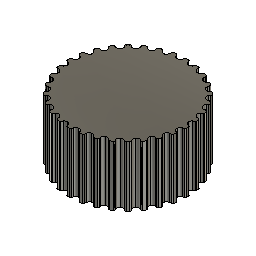
gear_32z (Autodesk Fusion 360 design; units mm, degrees)
Autodesk Fusion 360 part; units mm, degrees
sketch "Sketch1" plane through (0, 0, 0) normal (0, 0, 1) x (1, 0, 0) in component "gt2 pulley"
  circle A0 centre (0, 0) radius 10.1859 construction
  circle A1 centre (0, 0) radius 9.1819 construction
  line L0 (0, 0) -> (0, 10.1859) construction
  line L1 (0, 0) -> (0.9984, 10.1369) construction
  line L2 (0, 0) -> (1.4098, 10.0879) construction
  circle A2 centre (0, 0) radius 9.9319 construction
  arc A3 (0.3759, 9.7867) -> (0.4302, 9.5076) centre (1.3746, 9.8363) ccw
  circle A4 centre (0, 0) radius 9.7819 construction
  arc A5 (0.2295, 9.9293) -> (0, 9.9319) centre (0, 0) ccw
  arc A6 (0.3759, 9.7867) -> (0.2295, 9.9293) centre (0.2261, 9.7793) ccw
  arc A7 (0.4302, 9.5076) -> (0.9, 9.1377) centre (0.9544, 9.69) ccw
  arc A8 (0, 9.9319) -> (-0.2295, 9.9293) centre (0, 0) ccw
  arc A9 (-0.2295, 9.9293) -> (-0.3759, 9.7867) centre (-0.2261, 9.7793) ccw
  arc A10 (-0.4302, 9.5076) -> (-0.3759, 9.7867) centre (-1.3746, 9.8363) ccw
  arc A11 (-0.9002, 9.1377) -> (-0.4302, 9.5076) centre (-0.9544, 9.69) ccw
  arc A12 (0.9, 9.1377) -> (-0.9, 9.1377) centre (0, 0) ccw
  point P0 (1.3746, 9.8363)
  point P1 (0, 9.9319)
  dimension "d18" = 20.3718
  dimension "d19" = 5.625
  dimension "d22" = 1.004
  dimension "d24" = 0.75
  dimension "d26" = 1
  dimension "d27" = 0.15
  dimension "d28" = 0.15
  dimension "d47" = 0.555
  dimension "d52" = 3.812
  constraint coincident A0.centre A1.centre
  constraint coincident A0 L0.end
  constraint vertical L0
  constraint coincident A0 L1.end
  constraint coincident A0 L2.end
  constraint concentric A1 A2
  constraint coincident A1 A7.end
  constraint coincident L1 A7.end
  constraint coincident A2 P0
  constraint coincident L2 P0
  constraint coincident P0 A3.centre
  constraint coincident A2 P1
  constraint coincident L0 P1
  constraint concentric A2 A4
  constraint coincident P1 A5.end
  constraint coincident A4 A6.centre
  constraint coincident A3.start A6.start
  constraint tangent A3 A6
  constraint tangent A3 A7
  constraint symmetric L0 A7.end A12.end
  constraint symmetric L0 A3.start A9.end
  constraint symmetric L0 A3.end A10.start
  constraint symmetric L0 A3 A10
  constraint symmetric L0 A5.start A8.end
  constraint symmetric L0 P1 A5.end
  constraint symmetric L0 A5 A8
  constraint symmetric L0 A6 A9
  constraint symmetric L0 A7 A11
  constraint coincident A1 A11.start
  constraint tangent A1 A7
  constraint coincident L1 A7.centre
  measures "d18" diameter of A0
  measures "d19" angle of L0 L1
  measures "d22" distance of A0 A1
  measures "d24" distance of A1 A2
  measures "d26" radius of A3
  measures "d27" distance of A2 A4
  measures "d28" radius of A6
  measures "d47" radius of A7
extrude "Extrude1" add sketch "Sketch1" along normal blind 10 makes body 1
pattern_circular "C-Pattern1" count 32 over 360 about axis through (0, 0, 1.75) along (0, 0, 1) of bodies 1 makes body 2 at (-1.0991, 9.1159, 6.6667) makes body 3 at (-2.8564, 8.7263, 6.6667) makes body 4 at (-4.504, 8.0014, 6.6667) makes body 5 at (-5.9784, 6.9689, 6.6667) makes body 6 at (-7.5784, 5.1841, 6.6667) makes body 7 at (-8.4442, 3.606, 6.6667) makes body 8 at (-8.9854, 1.8893, 6.6667) makes body 9 at (-9.1551, -0.7007, 6.6667) makes body 10 at (-9.0245, -1.6931, 6.6667) makes body 11 at (-8.7263, -2.8564, 6.6667) makes body 12 at (-7.223, -5.6689, 6.6667) makes body 13 at (-6.9689, -5.9784, 6.6667) makes body 14 at (-4.5038, -8.0015, 6.6667) makes body 15 at (-3.606, -8.4442, 6.6667) makes body 16 at (-1.8893, -8.9854, 6.6667) makes body 17 at (0.7007, -9.1551, 6.6667) makes body 18 at (1.6931, -9.0245, 6.6667) makes body 19 at (2.8564, -8.7263, 6.6667) makes body 20 at (5.1843, -7.5783, 6.6667) makes body 21 at (6.9691, -5.9782, 6.6667) makes body 22 at (7.5784, -5.1841, 6.6667) makes body 23 at (8.1902, -4.1506, 6.6667) makes body 24 at (8.9854, -1.8893, 6.6667) makes body 25 at (9.1551, 0.7007, 6.6667) makes body 26 at (9.1159, 1.0991, 6.6667) makes body 27 at (8.7263, 2.8564, 6.6667) makes body 28 at (7.223, 5.6689, 6.6667) makes body 29 at (6.9689, 5.9784, 6.6667) makes body 30 at (5.1841, 7.5784, 6.6667) makes body 31 at (3.606, 8.4442, 6.6667) makes body 32 at (1.8893, 8.9854, 6.6667)
sketch "Sketch2" plane through (0, 0, 10) normal (0, 0, 1) x (-1, 0, 0)
  arc A0 (-9.672, -1.5406) -> (-9.7832, -1.712) centre (-9.6355, -1.6861) ccw
  arc A1 (-9.7832, -1.712) -> (-9.6937, -2.1622) centre (0, 0) ccw
  arc A2 (-9.6937, -2.1622) -> (-9.5254, -2.278) centre (-9.5473, -2.1296) ccw
  arc A3 (-9.241, -2.2768) -> (-9.5254, -2.278) centre (-9.3791, -3.2672) ccw
  arc A4 (-8.7865, -2.6654) -> (-9.241, -2.2768) centre (-9.3176, -2.8265) ccw
  arc A5 (-9.1377, -0.9) -> (-8.7865, -2.6654) centre (0, 0) ccw
  arc A6 (-9.4088, -1.4329) -> (-9.1377, -0.9) centre (-9.69, -0.9544) ccw
  arc A7 (-9.672, -1.5406) -> (-9.4088, -1.4329) centre (-9.9155, -0.5707) ccw
  circle A8 centre (0, 0) radius 9.1819
  constraint concentric A1 A8
extrude "Extrude2" add sketch "Sketch2" against normal blind 10 contours A5 A8 bodies 1 2 3 4 5 6 7 8 9 10 11 12 13 14 15 16 17 18 19 20 21 22 23 24 25 26 27 28 29 30 31 32
extrude "Extrude4" [suppressed] in component "gt2 pulley"
pattern_circular "C-Pattern7" [suppressed] in component "gt2 pulley"
extrude "Extrude3" [suppressed] in component "gt2 pulley"
pattern_circular "C-Pattern6" [suppressed] in component "gt2 pulley"
extrude "Extrude2'" [suppressed] in component "gt2 pulley"
pattern_circular "C-Pattern5" [suppressed] in component "gt2 pulley"
extrude "Extrude1'" [suppressed] in component "gt2 pulley"
pattern_circular "C-Pattern4" [suppressed] in component "gt2 pulley"
pattern_circular "C-Pattern3" [suppressed] in component "gt2 pulley"
pattern_circular "C-Pattern2" [suppressed] in component "gt2 pulley"
pattern_circular "C-Pattern1'" [suppressed] in component "gt2 pulley"
copy_body "Body->Comp1" [suppressed] in component "Component"
copy_body "Body->Comp2" [suppressed] in component "Component'"
copy_body "Body->Comp3" [suppressed] in component "Component''"
copy_body "Body->Comp4" [suppressed] in component "Component'''"
copy_body "Body->Comp5" [suppressed] in component "Component''''"
copy_body "Body->Comp6" [suppressed] in component "Component'''''"
copy_body "Body->Comp7" [suppressed] in component "Component''''''"
copy_body "Body->Comp8" [suppressed] in component "Component'''''''"
copy_body "Body->Comp9" [suppressed] in component "Component''''''''"
copy_body "Body->Comp10" [suppressed] in component "Component'''''''''"
copy_body "Body->Comp11" [suppressed] in component "Component''''''''''"
copy_body "Body->Comp12" [suppressed] in component "Component'''''''''''"
copy_body "Body->Comp13" [suppressed] in component "Component''''''''''''"
copy_body "Body->Comp14" [suppressed] in component "Component'''''''''''''"
copy_body "Body->Comp15" [suppressed] in component "Component''''''''''''''"
copy_body "Body->Comp16" [suppressed] in component "Component'''''''''''''''"
copy_body "Body->Comp17" [suppressed] in component "Component''''''''''''''''"
copy_body "Body->Comp18" [suppressed] in component "Component'''''''''''''''''"
copy_body "Body->Comp19" [suppressed] in component "Component''''''''''''''''''"
copy_body "Body->Comp20" [suppressed] in component "Component'''''''''''''''''''"
component "gt2 pulley" placed x (1, 0, 0) y (0, 1, 0) z (0, 0, 1) at (0, 0, 0)
equation "NumTeeth = 32" comment "min 20"
equation "ToothPitch = 2 mm"
equation "PullyDia = NumTeeth * ToothPitch / PI"
equation "ToothAng = ( ( 360 / NumTeeth ) * 1 deg )"
equation "TransOffsetAngle = ToothAng * 0.2"
equation "Sholulder_Radius = 0.15 mm"
equation "Root_Radius = 0.555 mm"
equation "TransRadius = 1 mm"
equation "ToolHeight = 0.75 mm"
equation "PLD = 0.254 mm"
equation "d18 = PullyDia"
equation "d19 = ToothAng / 2"
equation "d22 = PLD + ToolHeight"
equation "d24 = ToolHeight"
equation "d26 = TransRadius"
equation "d27 = Sholulder_Radius"
equation "d31 = NumTeeth"
equation "d33 = NumTeeth"
equation "d35 = NumTeeth"
equation "d37 = NumTeeth"
equation "d41 = NumTeeth"
equation "d45 = NumTeeth"
equation "d47 = Root_Radius"
equation "d50 = NumTeeth"
